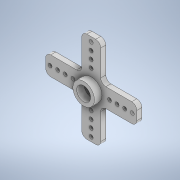
# Autodesk Inventor part: Звезда
Saved by Autodesk Inventor 2021 (Build 250183000, 183)
## iProperties
Created: 2022-07-09
Part Number: Звезда
Material: Типовые
Document SubType Name: Modeling
Designer: zvi20
Density: 1 g/cm^3
Appearance: По умолчанию
Author: zvi20
Autodesk Inventor part; units mm, degrees
ref_plane "YZ Plane" through (0, 0, 0) normal (1, 0, 0) x (0, 1, 0)
ref_plane "XZ Plane" through (0, 0, 0) normal (0, 1, 0) x (-1, 0, 0)
ref_plane "XY Plane" through (0, 0, 0) normal (0, 0, 1) x (1, 0, 0)
sketch "Эскиз1" plane through (0, 0, 0) normal (0, 0, 1) x (1, 0, 0)
  line L0 (83.9845, -81.4877) -> (83.9845, -84.9877)
  line L1 (47.9845, -84.9877) -> (47.9845, -81.4877)
  line L2 (64.2345, -65.2377) -> (67.7345, -65.2377)
  line L3 (67.7345, -101.2377) -> (64.2345, -101.2377)
  circle A0 centre (49.7345, -83.2377) radius 0.75
  circle A1 centre (52.7345, -83.2377) radius 0.75
  circle A2 centre (55.7345, -83.2377) radius 0.75
  circle A3 centre (58.7345, -83.2377) radius 0.75
  circle A4 centre (82.2345, -83.2377) radius 0.75
  circle A5 centre (79.2345, -83.2377) radius 0.75
  circle A6 centre (76.2345, -83.2377) radius 0.75
  circle A7 centre (73.2345, -83.2377) radius 0.75
  circle A8 centre (65.9845, -99.4877) radius 0.75
  circle A9 centre (65.9845, -96.4877) radius 0.75
  circle A10 centre (65.9845, -93.4877) radius 0.75
  circle A11 centre (65.9845, -90.4877) radius 0.75
  circle A12 centre (65.9845, -66.9877) radius 0.75
  circle A13 centre (65.9845, -69.9877) radius 0.75
  circle A14 centre (65.9845, -72.9877) radius 0.75
  circle A15 centre (65.9845, -75.9877) radius 0.75
  line L4 (49.9845, -79.4877) -> (60.2345, -79.4877)
  line L5 (71.7345, -79.4877) -> (81.9845, -79.4877)
  line L6 (62.2345, -99.2377) -> (62.2345, -88.9877)
  line L7 (62.2345, -77.4877) -> (62.2345, -67.2377)
  line L8 (81.9845, -86.9877) -> (71.7345, -86.9877)
  line L9 (60.2345, -86.9877) -> (49.9845, -86.9877)
  line L10 (69.7345, -67.2377) -> (69.7345, -77.4877)
  line L11 (69.7345, -88.9877) -> (69.7345, -99.2377)
  circle A16 centre (65.9845, -83.2377) radius 4.25
  circle A17 centre (65.9845, -83.2377) radius 2.75
  arc A18 (60.2345, -79.4877) -> (62.2345, -77.4877) centre (60.2345, -77.4877) ccw
  arc A19 (62.2345, -88.9877) -> (60.2345, -86.9877) centre (60.2345, -88.9877) ccw
  arc A20 (71.7345, -86.9877) -> (69.7345, -88.9877) centre (71.7345, -88.9877) ccw
  arc A21 (69.7345, -77.4877) -> (71.7345, -79.4877) centre (71.7345, -77.4877) ccw
  arc A22 (83.9845, -81.4877) -> (81.9845, -79.4877) centre (81.9845, -81.4877) ccw
  arc A23 (81.9845, -86.9877) -> (83.9845, -84.9877) centre (81.9845, -84.9877) ccw
  arc A24 (69.7345, -67.2377) -> (67.7345, -65.2377) centre (67.7345, -67.2377) ccw
  arc A25 (64.2345, -65.2377) -> (62.2345, -67.2377) centre (64.2345, -67.2377) ccw
  arc A26 (49.9845, -79.4877) -> (47.9845, -81.4877) centre (49.9845, -81.4877) ccw
  arc A27 (47.9845, -84.9877) -> (49.9845, -86.9877) centre (49.9845, -84.9877) ccw
  arc A28 (62.2345, -99.2377) -> (64.2345, -101.2377) centre (64.2345, -99.2377) ccw
  arc A29 (67.7345, -101.2377) -> (69.7345, -99.2377) centre (67.7345, -99.2377) ccw
  circle A30 centre (65.9845, -83.2377) radius 1.5
  point P0 (0, 0)
  point P1 (83.9845, -79.4877)
  point P2 (83.9845, -86.9877)
  point P3 (62.2345, -65.2377)
  point P4 (69.7345, -65.2377)
  point P5 (69.7345, -101.2377)
  point P6 (62.2345, -101.2377)
  dimension "d4" = 7.5
  dimension "d6" = 7.5
  dimension "d7" = 7.5
  dimension "d9" = 1.5
  dimension "d11" = 1.5
  dimension "d13" = 1.5
  dimension "d15" = 1.5
  dimension "d17" = 1.5
  dimension "d19" = 1.5
  dimension "d21" = 1.5
  dimension "d23" = 1.5
  dimension "d24" = 8.5
  dimension "d25" = 5.5
  dimension "d26" = 2
  dimension "d27" = 3
  constraints: 31 centre point, 24 end point, 24 point on circle, 24 tangent, 12 point on line, 11 equal radius, 4 perpendicular, 2 coincident, 2 vertical
  measures "d4" distance of point (83.985, -79.488) point (83.985, -86.988)
  measures "d6" distance of point (62.235, -65.238) point (69.735, -65.238)
  measures "d7" distance of point (69.735, -101.238) point (62.235, -101.238)
  measures "d9" diameter of A0
  measures "d11" diameter of A1
  measures "d13" diameter of A2
  measures "d15" diameter of A3
  measures "d17" diameter of A8
  measures "d19" diameter of A9
  measures "d21" diameter of A10
  measures "d23" diameter of A11
  measures "d24" diameter of A16
  measures "d25" diameter of A17
  measures "d26" radius of A18
  measures "d27" diameter of A30
extrude "Выдавливание1" add sketch "Эскиз1" along normal blind 2 contours L0 A23 L8 A20 L11 A29 L3 A28 L6 A19 L9 A27 L1 A26 L4 A18 L7 A25 L2 A24 L10 A21 L5 A22
extrude "Выдавливание2" add sketch "Эскиз1" along normal blind 5 contours A16
extrude "Выдавливание3" add sketch "Эскиз1" along normal blind 2 contours A17
